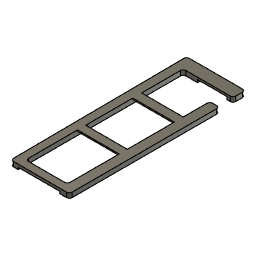
Calage_plaques (Autodesk Fusion 360 design; units mm, degrees)
Autodesk Fusion 360 part; units mm, degrees
sketch "Sketch1" plane through (0, 0, 0) normal (0, 1, 0) x (1, 0, 0)
  line L0 (15, 42) -> (15, -58.5)
  line L1 (13, -60.5) -> (-13.5, -60.5)
  line L2 (-15.5, -58.5) -> (-15.5, 53)
  line L3 (-13.5, 55) -> (19, 55)
  line L4 (21, 57) -> (21, 62)
  line L5 (19, 64) -> (-19.9844, 64)
  line L6 (-21.9844, 61.9844) -> (-20.9999, -64.0156)
  line L7 (-19, -66) -> (20, -66)
  line L8 (22, -64) -> (22, 42)
  line L9 (20, 44) -> (17, 44)
  arc A0 (22, 42) -> (20, 44) centre (20, 42) ccw
  arc A1 (17, 44) -> (15, 42) centre (17, 42) ccw
  arc A2 (20, -66) -> (22, -64) centre (20, -64) ccw
  arc A3 (13, -60.5) -> (15, -58.5) centre (13, -58.5) ccw
  arc A4 (-20.9999, -64.0156) -> (-19, -66) centre (-19, -64) ccw
  arc A5 (-15.5, -58.5) -> (-13.5, -60.5) centre (-13.5, -58.5) ccw
  arc A6 (-13.5, 55) -> (-15.5, 53) centre (-13.5, 53) ccw
  arc A7 (19, 55) -> (21, 57) centre (19, 57) ccw
  arc A8 (21, 62) -> (19, 64) centre (19, 62) ccw
  arc A9 (-19.9844, 64) -> (-21.9844, 61.9844) centre (-19.9844, 62) ccw
  dimension "d1" = 2
  constraint vertical L0
  constraint perpendicular L0 L1
  constraint perpendicular L1 L2
  constraint perpendicular L2 L3
  constraint perpendicular L1 L4
  constraint perpendicular L4 L5
  constraint perpendicular L4 L7
  constraint perpendicular L7 L8
  constraint perpendicular L0 L9
  constraint tangent L8 A0
  constraint tangent L9 A0
  constraint tangent L0 A1
  constraint tangent L9 A1
  constraint equal A0 A1
  constraint tangent L7 A2
  constraint tangent L8 A2
  constraint equal A0 A2
  constraint tangent L0 A3
  constraint tangent L1 A3
  constraint equal A0 A3
  constraint tangent L6 A4
  constraint tangent L7 A4
  constraint equal A0 A4
  constraint tangent L1 A5
  constraint tangent L2 A5
  constraint equal A0 A5
  constraint tangent L2 A6
  constraint tangent L3 A6
  constraint equal A0 A6
  constraint tangent L3 A7
  constraint tangent L4 A7
  constraint equal A0 A7
  constraint tangent L4 A8
  constraint tangent L5 A8
  constraint equal A0 A8
  constraint tangent L5 A9
  constraint tangent L6 A9
  constraint equal A0 A9
  measures "d1" radius of A0
extrude "Extrude1" add sketch "Sketch1" along normal blind 3.5
sketch "Sketch2" plane through (0, 3.5, 0) normal (0, 1, 0) x (-1, 0, 0)
  line L0 (13.5, -55) -> (-19, -55)
  arc A0 (-19, -55) -> (-21, -57) centre (-19, -57) ccw
  line L1 (-21, -57) -> (-21, -62)
  arc A1 (-21, -62) -> (-19, -64) centre (-19, -62) ccw
  line L2 (-19, -64) -> (19.9844, -64)
  arc A2 (19.9844, -64) -> (21.9844, -61.9844) centre (19.9844, -62) ccw
  line L3 (21.9844, -61.9844) -> (20.9999, 64.0156)
  arc A3 (20.9999, 64.0156) -> (19, 66) centre (19, 64) ccw
  line L4 (19, 66) -> (-20, 66)
  arc A4 (-20, 66) -> (-22, 64) centre (-20, 64) ccw
  line L5 (-22, 64) -> (-22, -42)
  arc A5 (-22, -42) -> (-20, -44) centre (-20, -42) ccw
  line L6 (-20, -44) -> (-17, -44)
  arc A6 (-17, -44) -> (-15, -42) centre (-17, -42) ccw
  line L7 (-15, -42) -> (-15, 58.5)
  arc A7 (-13, 60.5) -> (-15, 58.5) centre (-13, 58.5) ccw
  line L8 (-13, 60.5) -> (13.5, 60.5)
  arc A8 (15.5, 58.5) -> (13.5, 60.5) centre (13.5, 58.5) ccw
  line L9 (15.5, 58.5) -> (15.5, -53)
  arc A9 (13.5, -55) -> (15.5, -53) centre (13.5, -53) ccw
  line L10 (-14.988, 67.5) -> (15.5, 67.5)
  line L11 (15.5, 67.5) -> (15.5, 58.5)
  line L12 (15.5, 58.5) -> (-14.988, 58.5)
  line L13 (-14.988, 58.5) -> (-14.988, 67.5)
  constraint horizontal L10
  constraint vertical L11
  constraint horizontal L12
  constraint vertical L13
  constraint coincident A8.start L9.start
sketch "Sketch3" plane through (0, 0, 0) normal (0, -1, 0) x (1, 0, 0)
  line L0 (19, -55) -> (-13.5, -55)
  arc A0 (-15.5, -53) -> (-13.5, -55) centre (-13.5, -53) ccw
  line L1 (-15.5, -53) -> (-15.5, 58.5)
  arc A1 (-13.5, 60.5) -> (-15.5, 58.5) centre (-13.5, 58.5) ccw
  line L2 (-13.5, 60.5) -> (13, 60.5)
  arc A2 (15, 58.5) -> (13, 60.5) centre (13, 58.5) ccw
  line L3 (15, 58.5) -> (15, -42)
  arc A3 (15, -42) -> (17, -44) centre (17, -42) ccw
  line L4 (17, -44) -> (20, -44)
  arc A4 (20, -44) -> (22, -42) centre (20, -42) ccw
  line L5 (22, -42) -> (22, 64)
  arc A5 (22, 64) -> (20, 66) centre (20, 64) ccw
  line L6 (20, 66) -> (-19, 66)
  arc A6 (-19, 66) -> (-20.9999, 64.0156) centre (-19, 64) ccw
  line L7 (-20.9999, 64.0156) -> (-21.9844, -61.9844)
  arc A7 (-21.9844, -61.9844) -> (-19.9844, -64) centre (-19.9844, -62) ccw
  line L8 (-19.9844, -64) -> (19, -64)
  arc A8 (19, -64) -> (21, -62) centre (19, -62) ccw
  line L9 (21, -62) -> (21, -57)
  arc A9 (21, -57) -> (19, -55) centre (19, -57) ccw
  line L10 (-15.5, 51.9243) -> (14.988, 51.9243)
  line L11 (14.988, 51.9243) -> (14.988, 76)
  line L12 (14.988, 76) -> (-15.5, 76)
  line L13 (-15.5, 76) -> (-15.5, 51.9243)
  constraint horizontal L10
  constraint vertical L11
  constraint horizontal L12
  constraint vertical L13
  constraint coincident L1 L10.start
extrude "Extrude3" cut sketch "Sketch3" against normal blind 1.5 contours A1 L2 A2 L6 L11 L13
sketch "Sketch4" plane through (0, 3.5, 0) normal (0, 1, 0) x (-1, 0, 0)
  line L0 (13.5, -55) -> (-19, -55)
  arc A0 (-19, -55) -> (-21, -57) centre (-19, -57) ccw
  line L1 (-21, -57) -> (-21, -62)
  arc A1 (-21, -62) -> (-19, -64) centre (-19, -62) ccw
  line L2 (-19, -64) -> (19.9844, -64)
  arc A2 (19.9844, -64) -> (21.9844, -61.9844) centre (19.9844, -62) ccw
  line L3 (21.9844, -61.9844) -> (20.9999, 64.0156)
  arc A3 (20.9999, 64.0156) -> (19, 66) centre (19, 64) ccw
  line L4 (19, 66) -> (-20, 66)
  arc A4 (-20, 66) -> (-22, 64) centre (-20, 64) ccw
  line L5 (-22, 64) -> (-22, -42)
  arc A5 (-22, -42) -> (-20, -44) centre (-20, -42) ccw
  line L6 (-20, -44) -> (-17, -44)
  arc A6 (-17, -44) -> (-15, -42) centre (-17, -42) ccw
  line L7 (-15, -42) -> (-15, 58.5)
  arc A7 (-13, 60.5) -> (-15, 58.5) centre (-13, 58.5) ccw
  line L8 (-13, 60.5) -> (13.5, 60.5)
  arc A8 (15.5, 58.5) -> (13.5, 60.5) centre (13.5, 58.5) ccw
  line L9 (15.5, 58.5) -> (15.5, -53)
  arc A9 (13.5, -55) -> (15.5, -53) centre (13.5, -53) ccw
  line L10 (-15, -24.5) -> (17.4682, -24.5)
  line L11 (17.4682, -24.5) -> (17.4682, -18)
  line L12 (17.4682, -18) -> (-15, -18)
  line L13 (-15, -18) -> (-15, -24.5)
  line L14 (-15, 16.5) -> (17, 16.5)
  line L15 (17, 16.5) -> (17, 22.5)
  line L16 (17, 22.5) -> (-15, 22.5)
  line L17 (-15, 22.5) -> (-15, 16.5)
  line L18 (-13, 60.5) -> (13.5, 60.5)
  line L19 (-16.3717, -55) -> (5.5, -55)
  line L20 (5.5, -55) -> (5.5, -64)
  line L21 (5.5, -64) -> (-16.3717, -64)
  line L22 (-16.3717, -64) -> (-16.3717, -55)
  dimension "d10" = 6.5
  dimension "d11" = 6
  dimension "d12" = 38
  dimension "d13" = 78.5
  constraint horizontal L10
  constraint vertical L11
  constraint horizontal L12
  constraint vertical L13
  constraint coincident L7 L10.start
  constraint horizontal L14
  constraint vertical L15
  constraint horizontal L16
  constraint vertical L17
  constraint coincident L7 L14.start
  constraint horizontal L19
  constraint vertical L20
  constraint horizontal L21
  constraint vertical L22
  constraint coincident L2 L20.end
  constraint coincident L0 L19.start
  measures "d10" distance of L10 L12
  measures "d11" distance of L14 L16
  measures "d12" distance of L16 L18
  measures "d13" distance of L12 L18
extrude "Extrude4" add sketch "Sketch4" against normal blind 1 contours L7 L9 L10 L12 L13 | L7 L9 L14 L16 L17
sketch "Sketch5" plane through (0, 0, 0) normal (0, -1, 0) x (1, 0, 0)
  line L0 (-15.5, -53) -> (-15.5, 66)
  line L1 (-15.5, 66) -> (-19, 66)
  arc A0 (-19, 66) -> (-20.9999, 64.0156) centre (-19, 64) ccw
  line L2 (-20.9999, 64.0156) -> (-21.9844, -61.9844)
  arc A1 (-21.9844, -61.9844) -> (-19.9844, -64) centre (-19.9844, -62) ccw
  line L3 (-19.9844, -64) -> (19, -64)
  arc A2 (19, -64) -> (21, -62) centre (19, -62) ccw
  line L4 (21, -62) -> (21, -57)
  arc A3 (21, -57) -> (19, -55) centre (19, -57) ccw
  line L5 (19, -55) -> (-13.5, -55)
  arc A4 (-15.5, -53) -> (-13.5, -55) centre (-13.5, -53) ccw
  line L6 (16.5, -64) -> (-5, -64)
  line L7 (-5, -64) -> (-5, -55)
  line L8 (-5, -55) -> (16.5, -55)
  line L9 (16.5, -55) -> (16.5, -64)
  constraint horizontal L6
  constraint vertical L7
  constraint horizontal L8
  constraint vertical L9
  constraint coincident L5 L7.end
  constraint coincident L3 L6.start
extrude "Extrude5" cut sketch "Sketch5" against normal blind 2 contours L3 L5 L6 L7 L8 L9
